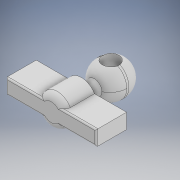
# Autodesk Inventor part: Luftregler2
Saved by Autodesk Inventor 2021 (Build 250183000, 183)
## iProperties
Created: 2021-10-22
Part Number: Luftregler2
Material: Generisch
Document SubType Name: Modeling
Designer: lukas
Density: 1 g/cm^3
Appearance: Vorgabe
Author: lukas
Autodesk Inventor part; units mm, degrees
ref_plane "YZ Plane" through (0, 0, 0) normal (1, 0, 0) x (0, 1, 0)
ref_plane "XY Plane" through (0, 0, 0) normal (0, 0, 1) x (1, 0, 0)
sketch "Skizze1" plane through (0, 0, 0) normal (0, 0, 1) x (1, 0, 0)
  line L0 (-21, 0) -> (21, 0) projected
  line L1 (0, -7) -> (0, 7) projected
  line L2 (-15, 2.5) -> (15, 2.5)
  line L3 (15, 2.5) -> (15, -2.5)
  line L4 (15, -2.5) -> (-15, -2.5)
  line L5 (-15, -2.5) -> (-15, 2.5)
  circle A0 centre (0, 0) radius 5
  point P0 (-4.3301, 2.5)
  point P1 (-4.3301, -2.5)
  point P2 (4.3301, -2.5)
  point P3 (4.3301, 2.5)
  dimension "d0" = 5
  dimension "d1" = 30
  dimension "d2" = 10
  constraints: 8 end point, 2 parallel, 1 centre point, 1 coincident, 1 horizontal, 1 perpendicular, 2 other
  measures "d0" distance between parallel lines of L2 L4
  measures "d1" distance between parallel lines of L3 L5
  measures "d2" diameter of A0
extrude "Extrusion1" add sketch "Skizze1" along normal blind 10
fillet "Rundung1" radius 2 2 edges at (0, 5, 10) (0, -5, 10)
fillet "Rundung2" radius 0.5 10 edges at (9.6651, -2.5, 10) (2.9942, -2.5, 10) (-9.6651, -2.5, 10) (-2.9942, -2.5, 10) (2.9942, 2.5, 10) (9.6651, 2.5, 10) (-2.9942, 2.5, 10) (-9.6651, 2.5, 10) (15, 0, 10) (-15, 0, 10)
sketch "Skizze2" plane through (0, 0, 0) normal (0, 0, -1) x (-1, 0, 0)
  circle A0 centre (0, 0) radius 2.5
  dimension "d7" = 5
  constraints: 1 centre point, 1 coincident
  measures "d7" diameter of A0
extrude "Extrusion2" add sketch "Skizze2" along normal blind 4.3
sketch "Skizze3" plane through (0, 0, -4.3) normal (0, 0, -1) x (-1, 0, 0)
  line L0 (5.7, -5.7) -> (-5.7, -5.7)
  line L1 (-5.7, -5.7) -> (-5.7, 5.7)
  line L2 (-5.7, 5.7) -> (5.7, 5.7)
  line L3 (5.7, 5.7) -> (5.7, -5.7)
  point P0 (0, 0)
  point P1 (0, 0)
  dimension "d11" = 11.4
  dimension "d12" = 11.4
  dimension "d13" = 5.7
  constraints: 8 end point, 2 parallel, 1 coincident, 1 horizontal, 1 perpendicular
  measures "d11" distance between parallel lines of L0 L2
  measures "d12" distance between parallel lines of L1 L3
  measures "d13" distance from line of point (0, 0) L2
extrude "Extrusion3" add sketch "Skizze3" along normal blind 11.4
fillet "Rundung3" radius 5.7 4 edges at (5.7, 5.7, -10) (-5.7, 5.7, -10) (5.7, -5.7, -10) (-5.7, -5.7, -10)
fillet "Rundung4" radius 5.6 8 edges at (-5.7, 0, -15.7) (-4.0305, -4.0305, -15.7) (-4.0305, 4.0305, -15.7) (0, -5.7, -15.7) (0, 5.7, -15.7) (4.0305, -4.0305, -15.7) (4.0305, 4.0305, -15.7) (5.7, 0, -15.7)
fillet "Rundung5" radius 5.6 8 edges at (-5.7, 0, -4.3) (-4.0305, -4.0305, -4.3) (-4.0305, 4.0305, -4.3) (0, -5.7, -4.3) (0, 5.7, -4.3) (4.0305, -4.0305, -4.3) (4.0305, 4.0305, -4.3) (5.7, 0, -4.3)
ref_plane "Arbeitsebene1" through (0, 5.7, 0) normal (0, 1, 0) x (-1, 0, 0)
sketch "Skizze4" plane through (0, 5.7, 0) normal (0, 1, 0) x (-1, 0, 0)
  circle A0 centre (0, -9.7096) radius 2.75
  point P0 (0, 0)
  point P1 (0, -9.3596)
  dimension "d20" = 0.35
  dimension "d21" = 5.5
  constraints: 1 centre point, 1 coincident
  measures "d20" distance of point (0, -9.36) point (0, -9.71)
  measures "d21" diameter of A0
extrude "Extrusion4" cut sketch "Skizze4" against normal blind 11.4
